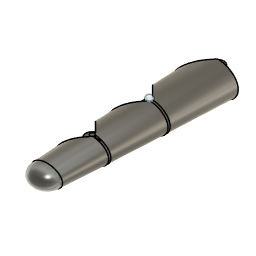
Assembly finger1 v3 (Autodesk Fusion 360 archive; units mm, degrees)
design "finger1.1"
Autodesk Fusion 360 part; units mm, degrees
note: some values were not read from the file. Set by a fixed rule: which face or edge a step refers to.
sketch "lower part" plane through (0, 0, 0) normal (0, 1, 0) x (1, 0, 0)
  ellipse E0 centre (0, 0) end of major axis (10, 0) minor radius 7.5
  line L0 (-10, 0) -> (10, 0) construction
  line L1 (0, -7.5) -> (0, 7.5) construction
  dimension "d1" = 20
  dimension "d2" = 15
  constraint coincident E0 L0.start
  constraint coincident E0 L0.end
  constraint coincident E0 L1.start
  constraint coincident E0 L1.end
  constraint coincident E0.centre origin
  constraint horizontal L0
  measures "d1" distance of E0
ref_plane "WorkPlane1" through (0, -30, 0) normal (0, 1, 0) x (1, 0, 0)
sketch "upper part" plane through (0, -30, 0) normal (0, 1, 0) x (1, 0, 0)
  ellipse E0 centre (0, 0) end of major axis (9, 0) minor radius 6.5
  line L0 (-9, 0) -> (9, 0) construction
  line L1 (0, -6.5) -> (0, 6.5) construction
  dimension "d4" = 18
  dimension "d5" = 13
  constraint coincident E0 L0.start
  constraint coincident E0 L0.end
  constraint coincident E0 L1.start
  constraint coincident E0 L1.end
  constraint coincident E0.centre origin
  constraint horizontal L0
  measures "d4" distance of E0
loft "Loft1" add profiles "upper part", "lower part" section 1 section 2 makes body 1
sketch "Sketch4" plane through (0, 0, 0) normal (0, 0, 1) x (1, 0, 0)
  line L0 (0, -30) -> (0, -29)
  line L1 (0, -29) -> (-17.6777, -11.3223)
  line L2 (0, -29) -> (25, -29) construction
  line L3 (0, 0) -> (0, -1)
  line L4 (0, -1) -> (-17.6777, -18.6777)
  line L5 (0, -1) -> (25, -1) construction
  line L6 (-9.7059, -10.7059) -> (-10, 0)
  line L7 (0, 0) -> (-10, 0)
  line L8 (-9.7059, -10.7059) -> (-16, 0)
  line L9 (-16, 0) -> (0, 0)
  line L10 (0, -30) -> (-11, -30)
  line L11 (-11, -30) -> (-9.3397, -19.6603)
  dimension "d6" = 1
  dimension "d7" = 135
  dimension "d8" = 25
  dimension "d9" = 135
  dimension "d10" = 25
  constraint vertical L0
  constraint horizontal L2
  constraint coincident L3.start L7.start
  constraint vertical L3
  constraint horizontal L5
  constraint coincident L4 L6.start
  constraint perpendicular L3 L7
  constraint perpendicular L3 L9
  constraint perpendicular L0 L10
  constraint coincident L1 L11.end
  measures "d6" distance of L0.start L0.end
  measures "d7" angle of L1 L2
  measures "d8" distance of L0.end L1.end
  measures "d9" angle of L4 L5
  measures "d10" distance of L3.end L4.end
extrude "Extrude1" cut sketch "Sketch4" along normal mid plane 80 bodies 1
sketch "Sketch5" plane through (0, 0, 0) normal (0, 0, 1) x (1, 0, 0)
  line L0 (0, 0) -> (0, 0.5)
  circle A0 centre (0, 0.5) radius 3
  line L1 (0, -30) -> (0, -30.5)
  circle A1 centre (0, -30.5) radius 3
  dimension "d13" = 0.5
  dimension "d14" = 6
  dimension "d15" = 0.5
  dimension "d16" = 6
  constraint coincident L0.start origin
  constraint vertical L0
  constraint coincident L0.end A0.centre
  constraint vertical L1
  constraint coincident L1.end A1.centre
  measures "d13" distance of L0.start L0.end
  measures "d14" diameter of A0
  measures "d15" distance of L1.start L1.end
  measures "d16" diameter of A1
extrude "Extrude2" add sketch "Sketch5" along normal mid plane 3 separate body contours A1 makes body 2
sketch "Sketch6" plane through (0, 0, 0) normal (0, 0, 1) x (1, 0, 0)
ref_plane "WorkPlane2" through (0, 0.5, 1.5) normal (0, 0, 1) x (1, 0, 0)
sketch "Sketch7" plane through (0, 0, 1.5) normal (0, 0, 1) x (1, 0, 0)
  circle A0 centre (0, 0.5) radius 3
  dimension "d20" = 6
  measures "d20" diameter of A0
extrude "Extrude3" add sketch "Sketch7" along normal blind 3 separate body makes body 3
ref_plane "WorkPlane3" through (0, 0.5, -1.5) normal (0, 0, 1) x (1, 0, 0)
sketch "Sketch8" plane through (0, 0, -1.5) normal (0, 0, 1) x (1, 0, 0)
  circle A0 centre (0, 0.5) radius 3
  dimension "d24" = 6
  measures "d24" diameter of A0
extrude "Extrude4" add sketch "Sketch8" against normal blind 3 separate body makes body 4
extrude "Extrude5" cut sketch "Sketch5" along normal mid plane 3 contours A0 bodies 1
sketch "Sketch9" plane through (0, 0, 0) normal (0, 0, 1) x (1, 0, 0)
  line L0 (0, 0) -> (0, 0.5)
  circle A0 centre (0, 0.5) radius 1
  line L1 (0, -30) -> (0, -30.5)
  circle A1 centre (0, -30.5) radius 1
  dimension "d30" = 2
  dimension "d32" = 2
  constraint coincident L0.start origin
  constraint vertical L0
  constraint coincident L0.end A0.centre
  constraint vertical L1
  constraint coincident L1.end A1.centre
  measures "d30" diameter of A0
  measures "d32" diameter of A1
extrude "Extrude6" cut sketch "Sketch9" along normal mid plane 40 contours A0 bodies 1 3 4
extrude "Extrude7" cut 1 faces at (-0.2669, -29.8198, -1.5) along direction (0, 0, -1) blind 3 on bodies 2 bodies 1
extrude "Extrude8" cut 1 faces at (-0.2669, -29.8198, 1.5) along direction (0, 0, 1) blind 3 on bodies 2 bodies 1
extrude "Extrude9" cut 1 faces at (-0.2669, -29.8198, -1.5) along direction (0, 0, 1) blind 2 on bodies 2 bodies 1 2
extrude "Extrude10" cut sketch "Sketch9" along normal mid plane 40 contours A1 bodies 1 2
extrude "Extrude11" add 1 faces at (2.3222, -30.649, 0.5) along direction (0, 0, -1) blind 2 on bodies 2 bodies 1 3 4 2
sketch "Sketch10" plane through (0, 0, 0) normal (0, 0, 1) x (1, 0, 0)
  line L0 (-10, 0) -> (-9, -30)
  line L1 (-9.8067, -5.8003) -> (-10.3064, -5.817)
  line L2 (-10.3064, -5.817) -> (-9.7052, -23.8517)
  line L3 (-9.7052, -23.8517) -> (-7.2066, -23.7684)
  line L4 (-10.3064, -5.817) -> (-7.8078, -5.7337)
  line L5 (-7.8078, -5.7337) -> (-7.2066, -23.7684)
  line L6 (-10.3064, -5.817) -> (-7.8078, -5.7337)
  arc A0 (-9.7052, -23.8517) -> (-7.2066, -23.7684) centre (-8.4559, -23.8101) ccw
  arc A1 (-9.7052, -23.8517) -> (-7.2066, -23.7684) centre (-8.4559, -23.8101) ccw
  dimension "d45" = 0.5
  dimension "d46" = 2.5
  dimension "d47" = 2.5
  constraint coincident L0 L1.start
  constraint perpendicular L0 L1
  constraint perpendicular L0 L3
  constraint parallel L0 L2
  constraint perpendicular L0 L4
  constraint parallel L2 L5
  constraint tangent L2 A0
  constraint tangent L2 A1
  measures "d45" distance of L1.start L1.end
  measures "d46" distance of L2.end L3.end
  measures "d47" distance of L1.end L4.end
extrude "Extrude12" cut sketch "Sketch10" along normal mid plane 2 contours L0 L3 L4 L5 L6 bodies 1
sketch "Sketch11" plane through (0, 0, 0) normal (0, 0, 1) x (1, 0, 0)
  line L0 (-8.876, -29.9959) -> (-9.876, 0.0041)
  line L1 (-9.0188, -25.7113) -> (-8.5191, -25.6946)
  line L2 (-8.5191, -25.6946) -> (-9.0025, -11.1937)
  line L3 (-9.5221, -10.6144) -> (-10.819, -10.6577)
  line L4 (-9.0025, -11.1937) -> (-8.003, -11.1604)
  line L5 (-8.003, -11.1604) -> (-7.6056, -23.0821)
  line L6 (-7.6056, -23.0821) -> (-8.5191, -25.6946)
  dimension "d50" = 0.5
  dimension "d51" = 1
  constraint coincident L0 L1.start
  constraint perpendicular L0 L1
  constraint parallel L0 L2
  constraint coincident L0 L3.start
  constraint perpendicular L0 L3
  constraint perpendicular L2 L4
  constraint perpendicular L4 L5
  measures "d50" distance of L1.start L1.end
  measures "d51" distance of L2.end L4.end
extrude "Extrude13" cut sketch "Sketch11" along normal mid plane 4 bodies 1
sketch "Sketch12" plane through (0, 0, 0) normal (0, 1, 0) x (1, 0, 0)
sketch "Sketch13" plane through (0, 0, 0) normal (0, 1, 0) x (1, 0, 0)
  ellipse E0 centre (0, 0) end of major axis (9, 0) minor radius 6.5
  line L0 (-9, 0) -> (9, 0) construction
  line L1 (0, -6.5) -> (0, 6.5) construction
  dimension "d54" = 18
  dimension "d55" = 13
  constraint coincident E0 L0.start
  constraint coincident E0 L0.end
  constraint coincident E0 L1.start
  constraint coincident E0 L1.end
  constraint coincident E0.centre origin
  constraint horizontal L0
  measures "d54" distance of E0
move_body "Move1" bodies 4 3 1 to x (1, 0, 0) y (0, 1, 0) z (0, 0, 1) at (51.617, 1.437, -0.2111)
sketch "Sketch14" plane through (0, 0, 0) normal (0, 1, 0) x (1, 0, 0)
ref_plane "WorkPlane4" through (0, -25, 0) normal (0, 1, 0) x (1, 0, 0)
sketch "Sketch15" plane through (0, -25, 0) normal (0, 1, 0) x (1, 0, 0)
  ellipse E0 centre (0, 0) end of major axis (-8, 0) minor radius 5.5
  line L0 (8, 0) -> (-8, 0) construction
  line L1 (0, 5.5) -> (0, -5.5) construction
  dimension "d57" = 16
  dimension "d58" = 11
  constraint coincident E0 L0.start
  constraint coincident E0 L0.end
  constraint coincident E0 L1.start
  constraint coincident E0 L1.end
  constraint coincident E0.centre origin
  constraint horizontal L0
  measures "d57" distance of E0
loft "Loft2" add profiles "Sketch15", "Sketch13" section 1 section 2 separate body makes body 5
sketch "Sketch16" plane through (0, 0, 0) normal (0, 0, 1) x (1, 0, 0)
  line L0 (0, -25) -> (0, -24)
  dimension "d59" = 1
  constraint vertical L0
  measures "d59" distance of L0.start L0.end
sketch "Sketch17" plane through (0, 0, 0) normal (0, 0, 1) x (1, 0, 0)
  line L0 (0, -25) -> (0, -24)
  line L1 (0, -24) -> (-14.1421, -9.8579)
  line L2 (0, -24) -> (20, -24) construction
  line L3 (0, 0) -> (0, -1)
  line L4 (0, -1) -> (-14.1421, -15.1421)
  line L5 (0, -1) -> (20, -1) construction
  line L6 (0, 0) -> (-11, 0)
  line L7 (-11, 0) -> (-10.3866, -11.3866)
  line L8 (0, -25) -> (-11.511, -25)
  line L9 (-11.511, -25) -> (-9.3937, -14.6063)
  dimension "d60" = 1
  dimension "d61" = 135
  dimension "d62" = 20
  dimension "d63" = 1
  dimension "d64" = 135
  dimension "d65" = 20
  constraint vertical L0
  constraint horizontal L2
  constraint coincident L3.start L6.start
  constraint vertical L3
  constraint horizontal L5
  constraint perpendicular L3 L6
  constraint coincident L4 L7.end
  constraint perpendicular L0 L8
  constraint coincident L1 L9.end
  measures "d60" distance of L0.start L0.end
  measures "d61" angle of L1 L2
  measures "d62" distance of L0.end L1.end
  measures "d63" distance of L3.start L3.end
  measures "d64" angle of L4 L5
  measures "d65" distance of L3.end L4.end
extrude "Extrude14" cut sketch "Sketch17" along normal mid plane 40 bodies 5
sketch "Sketch18" plane through (0, 0, 0) normal (0, 0, 1) x (1, 0, 0)
  line L0 (0, 0) -> (0, 0.5)
  circle A0 centre (0, 0.5) radius 3
  line L1 (0, -25) -> (0, -25.5)
  circle A1 centre (0, -25.5) radius 3
  dimension "d68" = 0.5
  dimension "d69" = 6
  dimension "d70" = 0.5
  dimension "d71" = 6
  constraint coincident L0.start origin
  constraint vertical L0
  constraint coincident L0.end A0.centre
  constraint vertical L1
  constraint coincident L1.end A1.centre
  measures "d68" distance of L0.start L0.end
  measures "d69" diameter of A0
  measures "d70" distance of L1.start L1.end
  measures "d71" diameter of A1
extrude "Extrude15" add sketch "Sketch18" along normal mid plane 3 separate body contours A1 makes body 6
extrude "Extrude16" cut 1 faces at (-0.5, -24.634, -1.5) along direction (0, 0, -1) blind 3 on bodies 6 bodies 5
extrude "Extrude17" cut 1 faces at (-0.5, -24.634, 1.5) along direction (0, 0, 1) blind 3 on bodies 6 bodies 5
extrude "Extrude18" cut sketch "Sketch18" along normal mid plane 3 contours A0 bodies 5
sketch "Sketch19" plane through (0, 0, 1.5) normal (0, 0, -1) x (1, 0, 0)
  line L0 (0, 0) -> (2.958, 0)
  arc A0 (2.958, 0) -> (-1.2343, 2.2343) centre (0, -0.5) ccw
  line L1 (-1.2343, 2.2343) -> (0, 1)
  line L2 (0, 1) -> (0, 0)
  line L3 (0, 0) -> (0, -0.5)
  circle A1 centre (0, -0.5) radius 3
  dimension "d80" = 0.5
  dimension "d81" = 6
  constraint coincident L0.start L2.end
  constraint perpendicular L0 L3
  constraint coincident A0.centre L3.end
  measures "d80" distance of L0.start A0.centre
  measures "d81" diameter of A1
extrude "Extrude19" add sketch "Sketch19" against normal blind 3 separate body makes body 7
sketch "Sketch20" plane through (0, 0, -1.5) normal (0, 0, 1) x (-1, 0, 0)
  line L0 (-2.958, 0) -> (0, 0)
  line L1 (0, 0) -> (0, 1)
  line L2 (0, 1) -> (1.2343, 2.2343)
  arc A0 (1.2343, 2.2343) -> (-2.958, 0) centre (0, -0.5) ccw
  line L3 (0, 0) -> (0, -0.5)
  circle A1 centre (0, -0.5) radius 3
  dimension "d84" = 0.5
  dimension "d85" = 6
  constraint coincident L0.end L1.start
  constraint perpendicular L0 L3
  constraint coincident A0.centre L3.end
  measures "d84" distance of L0.end A0.centre
  measures "d85" diameter of A1
extrude "Extrude20" add sketch "Sketch20" against normal blind 3 separate body makes body 8
sketch "Sketch21" plane through (0, 0, 4.5) normal (0, 0, 1) x (-1, 0, 0)
  circle A0 centre (0, -0.5) radius 3
  line L0 (0, 0) -> (0, -0.5)
  circle A1 centre (0, -0.5) radius 1
  line L1 (0, 25) -> (0, 25.5)
  circle A2 centre (0, 25.5) radius 1
  dimension "d88" = 0.5
  dimension "d89" = 2
  dimension "d90" = 0.5
  dimension "d91" = 2
  constraint coincident L0.start origin
  constraint vertical L0
  constraint coincident A0.centre L0.end
  constraint vertical L1
  constraint coincident L1.end A2.centre
  measures "d88" distance of L0.start A0.centre
  measures "d89" diameter of A1
  measures "d90" distance of L1.start L1.end
  measures "d91" diameter of A2
extrude "Extrude21" cut sketch "Sketch21" along normal mid plane 40 contours A1 | A2 bodies 5 6 7 8
sketch "Sketch22" plane through (0, 0, 0) normal (0, 0, 1) x (1, 0, 0)
sketch "Sketch23" plane through (0, 0, 0) normal (0, 1, 0) x (1, 0, 0)
sketch "Sketch24" plane through (0, -25, 0) normal (0, -1, 0) x (1, 0, 0)
  line L0 (0.866, 5.4677) -> (0.866, 4.5)
  line L1 (0.866, 4.5) -> (2.958, 4.5)
  line L2 (2.958, 4.5) -> (2.958, 1.5)
  line L3 (2.958, 1.5) -> (0.866, 1.5)
  line L4 (0.866, 1.5) -> (0.866, -1.5)
  line L5 (0.866, -1.5) -> (2.958, -1.5)
  line L6 (2.958, -1.5) -> (2.958, -4.5)
  line L7 (2.958, -4.5) -> (0.866, -4.5)
  line L8 (0.866, -4.5) -> (0.866, -5.4677)
  ellipse E0 centre (0, 0) end of major axis (-8, 0) minor radius 5.5 (0.866, -5.4677) -> (0.866, 5.4677) ccw
sketch "Sketch25" plane through (0, 0, 0) normal (0, 1, 0) x (1, 0, 0)
sketch "Sketch26" plane through (0, -25, 0) normal (0, -1, 0) x (1, 0, 0)
  ellipse E0 centre (0, 0) end of major axis (8, 0) minor radius 5.5
  line L0 (-8, 0) -> (8, 0) construction
  line L1 (0, -5.5) -> (0, 5.5) construction
  dimension "d94" = 16
  dimension "d95" = 11
  constraint coincident E0 L0.start
  constraint coincident E0 L0.end
  constraint coincident E0 L1.start
  constraint coincident E0 L1.end
  constraint coincident E0.centre origin
  constraint horizontal L0
  measures "d94" distance of E0
sketch "Sketch27" plane through (0, 0, 0) normal (0, 0, 1) x (1, 0, 0)
  line L0 (-8, -25) -> (-9, 0)
  line L1 (-8.2334, -19.164) -> (-8.733, -19.184)
  line L2 (-8.733, -19.184) -> (-9.2183, -7.0516)
  line L3 (-9.2183, -7.0516) -> (-6.7203, -6.9517)
  line L4 (-6.7203, -6.9517) -> (-6.2122, -19.6543)
  line L5 (-6.2122, -19.6543) -> (-10, -18)
  dimension "d96" = 0.5
  dimension "d97" = 2.5
  constraint coincident L0 L1.start
  constraint perpendicular L0 L1
  constraint perpendicular L1 L2
  constraint perpendicular L0 L3
  constraint perpendicular L3 L4
  measures "d96" distance of L1.start L1.end
  measures "d97" distance of L2.end L3.end
extrude "Extrude22" cut sketch "Sketch27" along normal mid plane 2 contours L0 L2 L3 L5 | L0 L3 L4 L5 bodies 5
sketch "Sketch28" plane through (0, 0, 0) normal (0, 0, 1) x (1, 0, 0)
  line L0 (-7.9485, -25.0019) -> (-8.9661, -0.0013)
  line L1 (-8.2232, -18.2539) -> (-7.7236, -18.2336)
  line L2 (-7.7236, -18.2336) -> (-8.0543, -10.1086)
  line L3 (-8.0543, -10.1086) -> (-7.0551, -10.0679)
  line L4 (-7.0551, -10.0679) -> (-6.6722, -19.477)
  line L5 (-6.6722, -19.477) -> (-9.7192, -14.7725)
  dimension "d100" = 0.5
  dimension "d101" = 1
  constraint coincident L0 L1.start
  constraint perpendicular L0 L1
  constraint perpendicular L1 L2
  constraint perpendicular L2 L3
  constraint perpendicular L3 L4
  measures "d100" distance of L1.start L1.end
  measures "d101" distance of L2.end L3.end
extrude "Extrude23" cut sketch "Sketch28" along normal mid plane 4 contours L2 L3 L4 L5 bodies 5
move_body "Move2" bodies 6 5 8 7 to x (1, 0, 0) y (0, 1, 0) z (0, 0, 1) at (-33.9665, 0, 4.1294)
sketch "Sketch29" plane through (0, 0, 0) normal (0, 1, 0) x (1, 0, 0)
  ellipse E0 centre (0, 0) end of major axis (8, 0) minor radius 5.5
  line L0 (-8, 0) -> (8, 0) construction
  line L1 (0, -5.5) -> (0, 5.5) construction
  dimension "d104" = 16
  dimension "d105" = 11
  constraint coincident E0 L0.start
  constraint coincident E0 L0.end
  constraint coincident E0 L1.start
  constraint coincident E0 L1.end
  constraint coincident E0.centre origin
  constraint horizontal L0
  measures "d104" distance of E0
ref_plane "WorkPlane5" through (0, -20, 0) normal (0, 1, 0) x (1, 0, 0)
sketch "Sketch30" plane through (0, -20, 0) normal (0, 1, 0) x (1, 0, 0)
  ellipse E0 centre (0, 0) end of major axis (7, 0) minor radius 4.5
  line L0 (-7, 0) -> (7, 0) construction
  line L1 (0, -4.5) -> (0, 4.5) construction
  dimension "d107" = 14
  dimension "d108" = 9
  constraint coincident E0 L0.start
  constraint coincident E0 L0.end
  constraint coincident E0 L1.start
  constraint coincident E0 L1.end
  constraint coincident E0.centre origin
  constraint horizontal L0
  measures "d107" distance of E0
loft "Loft3" add profiles "Sketch30", "Sketch29" section 1 section 2 separate body makes body 9
sketch "Sketch31" plane through (0, 0, 0) normal (0, 0, 1) x (1, 0, 0)
sketch "Sketch32" plane through (0, -20, 0) normal (0, -1, 0) x (1, 0, 0)
  ellipse E0 centre (0, 0) end of major axis (7, 0) minor radius 4.5
  line L0 (-7, 0) -> (7, 0)
  constraint coincident E0 L0.start
  constraint coincident E0 L0.end
  constraint horizontal L0
revolve "Revolve1" add sketch "Sketch32" angle 180 about axis through (-7, -20, 0) along (-1, 0, 0) contours E0 L0 picked at (-0.1497, -1.4969) bodies 9
sketch "Sketch33" plane through (0, 0, 0) normal (0, 0, 1) x (1, 0, 0)
sketch "Sketch34" plane through (0, 0, 0) normal (0, 0, 1) x (1, 0, 0)
  line L0 (0, 0) -> (0, 0.5)
  circle A0 centre (0, 0.5) radius 3
  dimension "d110" = 0.5
  dimension "d111" = 6
  constraint coincident L0.start origin
  constraint vertical L0
  constraint coincident L0.end A0.centre
  measures "d110" distance of L0.start L0.end
  measures "d111" diameter of A0
sketch "Sketch35" plane through (0, 0, 0) normal (0, 0, 1) x (1, 0, 0)
  line L0 (0, 0) -> (0, -1)
  line L1 (0, -1) -> (-14.1421, -15.1421)
  line L2 (0, -1) -> (20, -1) construction
  line L3 (-8, -9) -> (-11, 0)
  line L4 (-11, 0) -> (0, 0)
  dimension "d112" = 1
  dimension "d113" = 135
  dimension "d114" = 20
  constraint coincident L0.start L4.end
  constraint vertical L0
  constraint horizontal L2
  constraint coincident L1 L3.start
  constraint perpendicular L0 L4
  measures "d112" distance of L0.start L0.end
  measures "d113" angle of L1 L2
  measures "d114" distance of L0.end L1.end
extrude "Extrude24" cut sketch "Sketch35" along normal mid plane 40 bodies 9
sketch "Sketch36" plane through (0, 0, 0) normal (0, 0, 1) x (1, 0, 0)
  line L0 (0, 0) -> (0, 0.5)
  circle A0 centre (0, 0.5) radius 3
  dimension "d117" = 0.5
  dimension "d118" = 6
  constraint coincident L0.start origin
  constraint vertical L0
  constraint coincident L0.end A0.centre
  measures "d117" distance of L0.start L0.end
  measures "d118" diameter of A0
extrude "Extrude25" cut sketch "Sketch36" along normal mid plane 3 bodies 9
sketch "Sketch37" plane through (0, 0, 1.5) normal (0, 0, -1) x (1, 0, 0)
  line L0 (0, 0) -> (2.958, 0)
  arc A0 (2.958, 0) -> (-1.2343, 2.2343) centre (0, -0.5) ccw
  line L1 (-1.2343, 2.2343) -> (0, 1)
  line L2 (0, 1) -> (0, 0)
  line L3 (0, 0) -> (0, -0.5)
  circle A1 centre (0, -0.5) radius 3
  dimension "d121" = 0.5
  dimension "d122" = 6
  constraint coincident L0.start L2.end
  constraint perpendicular L0 L3
  constraint coincident A0.centre L3.end
  measures "d121" distance of L0.start A0.centre
  measures "d122" diameter of A1
extrude "Extrude26" add sketch "Sketch37" against normal blind 3 separate body makes body 10
sketch "Sketch38" plane through (0, 0, -1.5) normal (0, 0, 1) x (-1, 0, 0)
  line L0 (-2.958, 0) -> (0, 0)
  line L1 (0, 0) -> (0, 1)
  line L2 (0, 1) -> (1.2343, 2.2343)
  arc A0 (1.2343, 2.2343) -> (-2.958, 0) centre (0, -0.5) ccw
  line L3 (0, 0) -> (0, -0.5)
  circle A1 centre (0, -0.5) radius 3
  dimension "d125" = 0.5
  dimension "d126" = 6
  constraint coincident L0.end L1.start
  constraint perpendicular L0 L3
  constraint concentric A0 A1
  measures "d125" distance of L0.end A0.centre
  measures "d126" diameter of A1
extrude "Extrude27" add sketch "Sketch38" against normal blind 3 bodies 9
sketch "Sketch39" plane through (0, 0, -4.5) normal (0, 0, -1) x (1, 0, 0)
  line L0 (0, 1) -> (-1.2343, 2.2343)
  arc A0 (-1.2343, 2.2343) -> (2.958, 0) centre (0, -0.5) ccw
  line L1 (2.958, 0) -> (0, 0)
  line L2 (0, 0) -> (0, 1)
  circle A1 centre (0, -0.5) radius 1
  dimension "d129" = 2
  constraint concentric A0 A1
  measures "d129" diameter of A1
extrude "Extrude28" cut sketch "Sketch39" along normal mid plane 40 contours L1 L2 A1 | L1 L2 A1 bodies 9 10
sketch "Sketch40" plane through (0, 0, 0) normal (0, 1, 0) x (1, 0, 0)
sketch "Sketch41" plane through (0, -20, 0) normal (0, 1, 0) x (1, 0, 0)
  line L0 (0, 0) -> (0, -4.5)
  line L1 (0, 0) -> (0, 4.5)
  ellipse E0 centre (0, 0) end of major axis (7, 0) minor radius 4.5 (0, -4.5) -> (0, 4.5) ccw
  dimension "d132" = 14
  dimension "d133" = 9
  dimension "d134" = 4.5
  constraint coincident L0.start L1.start
  measures "d132" distance of E0
  measures "d134" distance of L0.start L1.end
revolve "Revolve2" add sketch "Sketch41" angle 180 about axis through (0, -20, 0) along (0, 0, -1) bodies 9
move_body "Move3" bodies 9 10 to x (1, 0, 0) y (0, 1, 0) z (0, 0, 1) at (-0.073, -49.9376, 2.4954)
sketch "Sketch42" plane through (0, 0, 0) normal (0, 0, 1) x (1, 0, 0)
  circle A0 centre (0, 0) radius 1
  dimension "d136" = 2
  constraint coincident A0.centre origin
  measures "d136" diameter of A0
extrude "Extrude29" add sketch "Sketch42" along normal mid plane 18 separate body makes body 11
move_body "Move4" bodies 11 to x (1, 0, 0) y (0, 1, 0) z (0, 0, 1) at (0, 10, 0)
sketch "Sketch43" plane through (0, 0, 0) normal (0, 0, 1) x (1, 0, 0)
  circle A0 centre (0, 0) radius 1
  dimension "d139" = 2
  constraint coincident A0.centre origin
  measures "d139" diameter of A0
extrude "Extrude30" add sketch "Sketch43" along normal mid plane 16 separate body makes body 12
move_face "MoveFace1" by (-5, 10, 0) 1 faces at (-0.3296, 0.5031, -8) on bodies 12
copy_body "Body->Comp1" bodies 3 removing the originals makes body 13 in component "Component"
copy_body "Body->Comp2" bodies 4 removing the originals makes body 14 in component "Component'"
copy_body "Body->Comp3" bodies 1 removing the originals makes body 15 in component "finger part 1"
copy_body "Body->Comp4" bodies 5 removing the originals makes body 16 in component "Component''"
copy_body "Body->Comp5" bodies 6 removing the originals makes body 17 in component "Component'''"
copy_body "Body->Comp6" bodies 7 removing the originals makes body 18 in component "Component''''"
copy_body "Body->Comp7" bodies 8 removing the originals makes body 19 in component "Component'''''"
copy_body "Body->Comp8" bodies 9 removing the originals makes body 20 in component "Component''''''"
copy_body "Body->Comp9" bodies 10 removing the originals makes body 21 in component "Component'''''''"
copy_body "Body->Comp10" bodies 11 removing the originals makes body 22 in component "Component''''''''"
copy_body "Body->Comp11" bodies 12 removing the originals makes body 23 in component "Component'''''''''"
combine "Combine1" operation add target body 21 tool bodies 20 in component "Component'''''''"
combine "Combine1'" operation add target body 16 tool bodies 19 18 in component "Component''"
combine "Combine1''" operation add target body 15 tool bodies 14 13 in component "finger part 1"
move_face "MoveFace1'" to x (1, 0, 0) y (0, 1, 0) z (0, 0, 1) at (-6.0421, -52.9106, -14.2185) 2 faces at (0.9988, 9.9502, 6) (0.9988, 9.9502, -6) on bodies 22 in component "Component''''''''"
delete_body "RemoveBody1" bodies 23 in component "Component'''''''''"
sketch "Sketch44" plane through (0, 0, 0) normal (0, 0, 1) x (1, 0, 0)
  circle A0 centre (0, 0) radius 1
  dimension "d142" = 2
  constraint coincident A0.centre origin
  measures "d142" diameter of A0
sketch "Sketch45" plane through (0, 0, 0) normal (0, 0, 1) x (1, 0, 0)
sketch "Sketch46" plane through (0, 0, 0) normal (0, 0, 1) x (1, 0, 0)
  circle A0 centre (0, 0) radius 1
  dimension "d145" = 2
  constraint coincident A0.centre origin
  measures "d145" diameter of A0
extrude "Extrude32" add sketch "Sketch46" along normal mid plane 10 separate body makes body 24
copy_body "Body->Comp12" bodies 24 removing the originals makes body 25 in component "Component''''''''''"
sketch "Sketch47" plane through (0, 0, 0) normal (0, 0, 1) x (1, 0, 0)
  circle A0 centre (0, 0) radius 1
  circle A1 centre (-9, -15) radius 1
  dimension "d148" = 2
  dimension "d149" = 2
  constraint coincident A0.centre origin
  measures "d148" diameter of A0
  measures "d149" diameter of A1
extrude "Extrude33" add sketch "Sketch47" along normal mid plane 11 separate body contours A0 makes body 26
copy_body "Body->Comp13" bodies 26 removing the originals makes body 27 in component "Component'''''''''''"
sketch "Sketch48" plane through (0, 0, 0) normal (0, 0, 1) x (1, 0, 0)
sketch "Sketch49" plane through (0, 0, 0) normal (0, 0, 1) x (1, 0, 0)
  circle A0 centre (0, 0) radius 1
  dimension "d152" = 2
  constraint coincident A0.centre origin
  measures "d152" diameter of A0
extrude "Extrude34" add sketch "Sketch49" along normal mid plane 13 separate body makes body 28
sketch "Sketch50" plane through (0, 0, 8.6294) normal (0, 0, 1) x (-1, 0, 0)
  line L0 (33.1005, 0) -> (31.0084, 0)
  arc A0 (31.0084, 0) -> (35.2008, 2.2343) centre (33.9665, -0.5) ccw
  line L1 (35.2008, 2.2343) -> (33.9665, 1)
  line L2 (33.9665, 1) -> (33.9665, 0.5)
  arc A1 (33.1005, 0) -> (33.9665, 0.5) centre (33.9665, -0.5) ccw
ref_plane "WorkPlane6" through (-34.1301, 0.9297, 10.6294) normal (0, 0, 1) x (-1, 0, 0)
sketch "Sketch51" plane through (0, 0, 10.6294) normal (0, 0, 1) x (1, 0, 0)
  circle A0 centre (-33.9552, 0.5401) radius 1
  dimension "d156" = 2
  measures "d156" diameter of A0
copy_body "Body->Comp14" bodies 28 removing the originals makes body 29 in component "Component''''''''''''"
component "Component" placed x (1, 0, 0) y (0, 1, 0) z (0, 0, 1) at (0, 0, 0)
component "Component'" placed x (1, 0, 0) y (0, 1, 0) z (0, 0, 1) at (0, 0, 0)
component "finger part 1" placed x (1, 0, 0) y (0, 1, 0) z (0, 0, 1) at (-85.5835, 29.563, 4.3405)
component "Component''" placed x (1, 0, 0) y (0, 1, 0) z (0, 0, 1) at (0, 0, 0)
component "Component'''" placed x (1, 0, 0) y (0, 1, 0) z (0, 0, 1) at (0, 0, 0)
component "Component''''" placed x (1, 0, 0) y (0, 1, 0) z (0, 0, 1) at (0, 0, 0)
component "Component'''''" placed x (1, 0, 0) y (0, 1, 0) z (0, 0, 1) at (0, 0, 0)
component "Component''''''" placed x (1, 0, 0) y (0, 1, 0) z (0, 0, 1) at (0, 0, 0)
component "Component'''''''" placed x (1, 0, 0) y (0, 1, 0) z (0, 0, 1) at (-33.8934, 23.9376, 1.634)
component "Component'''''''''" placed x (1, 0, 0) y (0, 1, 0) z (0, 0, 1) at (0, 0, 0)
component "Component'''''''''''" placed x (1, 0, 0) y (0, 1, 0) z (0, 0, 1) at (-33.9665, -25.5, 4.1544)
component "Component''''''''''''" placed x (1, 0, 0) y (0, 1, 0) z (0, 0, 1) at (0, 0, 0)
equation "d39 = 0 mm - 2.00 mm"
equation "d82 = 0 mm - 3.00 mm"
equation "d86 = 0 mm - 3.00 mm"
equation "d106 = 0 mm - 20.00 mm"
equation "d123 = 0 mm - 3.00 mm"
equation "d127 = 0 mm - 3.00 mm"
named bodies: "finger part 1"
